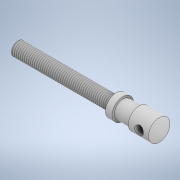
# Autodesk Inventor part: Parafuso1
Saved by Autodesk Inventor 2021 (Build 250183000, 183)
## iProperties
Created: 2022-02-15
Part Number: Parafuso1
Material: Genérico
Document SubType Name: Modeling
Designer: aluno
Density: 1 g/cm^3
Appearance: Padrão
Author: aluno
Autodesk Inventor part; units mm, degrees
ref_plane "YZ Plane" through (0, 0, 0) normal (1, 0, 0) x (0, 1, 0)
ref_plane "XZ Plane" through (0, 0, 0) normal (0, 1, 0) x (-1, 0, 0)
ref_plane "XY Plane" through (0, 0, 0) normal (0, 0, 1) x (1, 0, 0)
sketch "Esboço1" plane through (0, 0, 0) normal (0, 0, 1) x (1, 0, 0)
  line L0 (0, 0) -> (107, 0)
  line L1 (0, 0) -> (0, 5)
  line L2 (0, 5) -> (73, 5)
  line L3 (73, 5) -> (73, 8)
  line L4 (73, 8) -> (78, 8)
  line L5 (78, 8) -> (78, 6.5)
  line L6 (78, 6.5) -> (90, 6.5)
  line L7 (90, 6.5) -> (90, 8)
  line L8 (90, 8) -> (105, 8)
  arc A0 (107, 0) -> (105, 8) centre (90, 0) ccw
  dimension "d0" = 107
  dimension "d2" = 73
  dimension "d4" = 5
  dimension "d6" = 12
  dimension "d8" = 15
  dimension "d9" = 10
  dimension "d10" = 16
  dimension "d11" = 13
  dimension "d12" = 16
  constraints: 18 end point, 5 perpendicular, 2 horizontal, 2 point on circle, 2 vertical, 1 centre point, 1 point on line
  measures "d0" distance of L0.start L0.end
  measures "d2" distance of L1.end L2.end
  measures "d4" distance of L3.end L4.end
  measures "d6" distance of L5.end L6.end
  measures "d8" distance of L7.end L8.end
  measures "d9" diameter of L2 L0
  measures "d10" diameter of L4 L0
  measures "d11" diameter of L6 L0
  measures "d12" diameter of L8 L0
revolve "Revolução1" add sketch "Esboço1" angle 360 about axis through (0, 0, 0) along (1, 0, 0)
thread "Rosca1" size "M10x1.5" class "6g" standard "ISO Metric profile" full length
sketch "Esboço2" plane through (0, 0, 0) normal (0, 0, 1) x (1, 0, 0)
  circle A0 centre (98, 0) radius 3.25
  line L0 (0, -5) -> (0, 5) projected
  line L1 (0, 5) -> (73, 5) projected
  line L2 (73, 5) -> (73, 8) projected
  line L3 (73, 8) -> (78, 8) projected
  line L4 (78, 8) -> (78, 6.5) projected
  line L5 (78, 6.5) -> (90, 6.5) projected
  line L6 (90, 6.5) -> (90, 8) projected
  line L7 (90, 8) -> (105, 8) projected
  arc A1 (105, -8) -> (105, 8) centre (90, 0) ccw projected
  line L8 (105, -8) -> (90, -8) projected
  line L9 (90, -8) -> (90, -6.5) projected
  line L10 (90, -6.5) -> (78, -6.5) projected
  line L11 (78, -6.5) -> (78, -8) projected
  line L12 (78, -8) -> (73, -8) projected
  line L13 (73, -8) -> (73, -5) projected
  line L14 (73, -5) -> (0, -5) projected
  point P0 (0, 0)
  dimension "d16" = 6.5
  dimension "d17" = 7
  constraints: 1 centre point, 1 horizontal alignment
  measures "d16" diameter of A0
  measures "d17" horizontal distance of A0.centre L7.end
extrude "Extrusão1" cut sketch "Esboço2" along normal through all both and the other way through all contours A0
